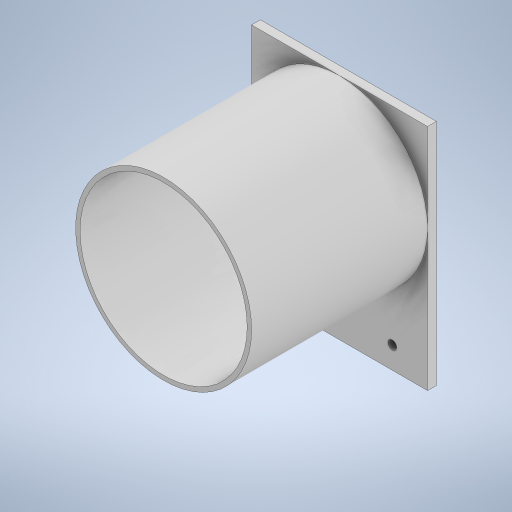
# Autodesk Inventor part: Reservoir
Saved by Autodesk Inventor 2024 (Build 280153000, 153)
## iProperties
Created: 2024-02-05
Part Number: Reservoir
Material: Generic
Document SubType Name: Modeling
Designer: Ramji Yadav
Density: 1 g/cm^3
Appearance: Default
Author: Ramji Yadav
Autodesk Inventor part; units mm, degrees
ref_plane "YZ Plane" through (0, 0, 0) normal (1, 0, 0) x (0, 1, 0)
ref_plane "XZ Plane" through (0, 0, 0) normal (0, 1, 0) x (-1, 0, 0)
ref_plane "XY Plane" through (0, 0, 0) normal (0, 0, 1) x (1, 0, 0)
sketch "Sketch1" plane through (0, 0, 0) normal (0, 0, 1) x (1, 0, 0)
  line L0 (0, 0) -> (100, 0)
  line L1 (100, 0) -> (100, 130)
  line L2 (100, 130) -> (0, 130)
  line L3 (0, 130) -> (0, 0)
  dimension "d0" = 100
  dimension "d1" = 130
  constraints: 8 end point, 2 parallel, 1 horizontal, 1 perpendicular
  measures "d0" distance of L2.end L1.end
  measures "d1" distance of L1.end L0.end
extrude "Extrusion1" add sketch "Sketch1" along normal blind 5
sketch "Sketch2" plane through (0, 0, 5) normal (0, 0, 1) x (1, 0, 0)
  line L0 (0, 130) -> (0, 0) projected
  line L1 (100, 130) -> (0, 130) projected
  line L2 (0, 0) -> (100, 0)
  line L3 (100, 0) -> (100, 130)
  line L4 (100, 130) -> (0, 130)
  line L5 (0, 130) -> (0, 0)
  circle A0 centre (50, 80) radius 50
  circle A1 centre (50, 80) radius 47.5
  dimension "d4" = 95
  constraints: 8 end point, 3 tangent, 2 centre point, 2 parallel, 1 coincident, 1 horizontal, 1 perpendicular
  measures "d4" diameter of A1
extrude "Extrusion2" add sketch "Sketch2" along normal blind 100 contours A0
sketch "Sketch3" plane through (0, 0, 5) normal (0, 0, 1) x (1, 0, 0)
  line L0 (100, 0) -> (100, 130) projected
  line L1 (0, 80) -> (0, 0) projected
  line L2 (100, 0) -> (0, 0)
  line L3 (0, 0) -> (0, 25)
  line L4 (0, 25) -> (100, 25)
  line L5 (100, 25) -> (100, 0)
  circle A0 centre (80, 12.5) radius 2.5
  circle A1 centre (20, 12.5) radius 2.5
  point P0 (0, 12.5)
  point P1 (100, 12.5)
  dimension "d7" = 25
  dimension "d8" = 5
  dimension "d9" = 5
  dimension "d10" = 20
  dimension "d11" = 20
  dimension "d12" = 12.5
  dimension "d13" = 12.5
  constraints: 8 end point, 2 centre point, 2 midpoint, 2 parallel, 1 horizontal, 1 perpendicular, 1 point on line
  measures "d7" distance of L2.end L3.end
  measures "d8" diameter of A0
  measures "d9" diameter of A1
  measures "d10" distance of point (0, 12.5) A1.centre
  measures "d11" distance of point (100, 12.5) A0.centre
  measures "d12" distance from line of L4 A1.centre
  measures "d13" distance from line of L4 A0.centre
extrude "Extrusion3" cut sketch "Sketch3" against normal blind 100 contours A0 | A1
thread "Thread1" size "M5x0.8" class "6H" standard "ANSI Metric M Profile" full length
thread "Thread2" size "M5x0.8" class "6H" standard "ANSI Metric M Profile" full length
body "Solid1"
